# Autodesk Inventor part: SWITCH-MOMENTARY-2SMD-4
Saved by Autodesk Inventor 2016 (Build 200138000, 138)
## iProperties
Created: 2016-04-08
Part Number: SWITCH-MOMENTARY-2SMD-4
Material: Generic
Document SubType Name: Modeling
Designer: Paschalis
Density: 1 g/cm^3
Appearance: TACTILE_SWITCH_TALL, SWITCH-MOMENTARY-2SMD-4
Author: Paschalis
Autodesk Inventor part; units mm, degrees
ref_plane "YZ Plane" through (0, 0, 0) normal (1, 0, 0) x (0, 1, 0)
ref_plane "XZ Plane" through (0, 0, 0) normal (0, 1, 0) x (-1, 0, 0)
ref_plane "XY Plane" through (0, 0, 0) normal (0, 0, 1) x (1, 0, 0)
sketch "TACTILE_SWITCH_TALL, SWITCH-MOMENTARY-2SMD-4_115" plane through (0, 0, 0) normal (0, 0, 1) x (1, 0, 0)
  line L0 (-3.127, 3) -> (3.127, 3)
  line L1 (3.127, 3) -> (3.127, -3.127)
  line L2 (3.127, -3.127) -> (-3.127, -3.127)
  line L3 (-3.127, -3.127) -> (-3.127, 3)
  constraints: 8 end point
extrude "Extrusion1" add sketch "TACTILE_SWITCH_TALL, SWITCH-MOMENTARY-2SMD-4_115" along normal blind 1
body "Solid1"
